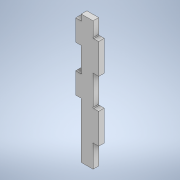
# Autodesk Inventor part: cover
Saved by Autodesk Inventor 2020 (Build 240168000, 168)
## iProperties
Created: 2019-12-19
Part Number: cover
Material: Générique
Document SubType Name: Modeling
Designer: damien
Density: 1 g/cm^3
Appearance: Par défaut
Author: damien
Autodesk Inventor part; units mm, degrees
ref_plane "YZ Plane" through (0, 0, 0) normal (1, 0, 0) x (0, 1, 0)
ref_plane "XZ Plane" through (0, 0, 0) normal (0, 1, 0) x (-1, 0, 0)
ref_plane "XY Plane" through (0, 0, 0) normal (0, 0, 1) x (1, 0, 0)
sketch "Esquisse3" plane through (0, 0, 0) normal (0, 0, 1) x (1, 0, 0)
  line L0 (38, -212.5) -> (-38, -212.5)
  line L1 (-38, -212.5) -> (-38, 212.5)
  line L2 (-38, 212.5) -> (38, 212.5)
  line L3 (38, 212.5) -> (38, -212.5)
  line L4 (38, -212.5) -> (-38, 212.5) construction
  line L5 (-38, -212.5) -> (38, 212.5) construction
  point P0 (0, 0)
  dimension "d20" = 76
  dimension "d21" = 425
  constraints: 12 end point, 2 midpoint, 2 parallel, 1 horizontal, 1 perpendicular
  measures "d20" distance of L0.start L0.end
  measures "d21" distance of L2.end L0.start
extrude "Extrusion3" add sketch "Esquisse3" along normal blind 18.55
sketch "Esquisse4" plane through (0, 0, 18.55) normal (0, 0, 1) x (1, 0, 0)
  line L0 (38, 212.5) -> (19.4, 212.5)
  line L1 (19.4, 212.5) -> (19.4, 162.4)
  line L2 (19.4, 162.4) -> (38, 162.4)
  line L3 (38, 162.4) -> (38, 212.5)
  line L4 (-38, -212.5) -> (38, -212.5) projected
  line L5 (38, -212.5) -> (19.4, -212.5)
  line L6 (19.4, -212.5) -> (19.4, -137.4)
  line L7 (19.4, -137.4) -> (38, -137.4)
  line L8 (38, -137.4) -> (38, -212.5)
  line L9 (38, -37.6) -> (19.4, -37.6)
  line L10 (19.4, -37.6) -> (19.4, 62.6)
  line L11 (19.4, 62.6) -> (38, 62.6)
  line L12 (38, 62.6) -> (38, -37.6)
  point P0 (0, 0)
  dimension "d24" = 75.1
  dimension "d25" = 50.1
  dimension "d27" = 100.2
  dimension "d29" = 99.8
  dimension "d30" = 99.8
  dimension "d31" = 18.6
  constraints: 24 end point, 6 parallel, 3 horizontal, 3 perpendicular, 2 collinear, 1 point on line
  measures "d24" distance of L5.end L6.end
  measures "d25" distance of L0.end L1.end
  measures "d27" distance of L9.end L10.end
  measures "d29" distance between parallel lines of L7 L9
  measures "d30" distance between parallel lines of L2 L11
  measures "d31" distance between parallel lines of L12 L10
extrude "Extrusion4" cut sketch "Esquisse4" against normal blind 18.55
sketch "Esquisse5" plane through (0, 0, 18.55) normal (0, 0, 1) x (1, 0, 0)
  line L0 (19.4, 212.5) -> (-38, 212.5) projected
  line L1 (-38, 212.5) -> (-19.45, 212.5)
  line L2 (-19.45, 212.5) -> (-19.45, 192.4)
  line L3 (-19.45, 192.4) -> (-38, 192.4)
  line L4 (-38, 192.4) -> (-38, 212.5)
  line L5 (-38, 212.5) -> (-38, -212.5) projected
  line L6 (-38, 122.5) -> (-19.45, 122.5)
  line L7 (-19.45, 122.5) -> (-19.45, 41)
  line L8 (-19.45, 41) -> (-38, 41)
  line L9 (-38, 41) -> (-38, 122.5)
  line L10 (-38, -28.9) -> (-19.45, -28.9)
  line L11 (-19.45, -28.9) -> (-19.45, -212.5)
  line L12 (-19.45, -212.5) -> (-38, -212.5)
  line L13 (-38, -212.5) -> (-38, -28.9)
  line L14 (-38, -212.5) -> (19.4, -212.5) projected
  point P0 (0, 0)
  point P1 (-38, 41)
  dimension "d34" = 20.1
  dimension "d35" = 18.55
  dimension "d37" = 69.9
  dimension "d38" = 81.5
  dimension "d39" = 69.9
  constraints: 24 end point, 6 parallel, 3 collinear, 3 horizontal, 3 perpendicular, 2 point on line
  measures "d34" distance of L3.end L0.end
  measures "d35" distance from line of L2 L3.end
  measures "d37" distance between parallel lines of L6 L3
  measures "d38" distance of L6.end L7.end
  measures "d39" distance between parallel lines of L10 L8
extrude "Extrusion5" cut sketch "Esquisse5" against normal blind 18.55
sketch "Esquisse6" plane through (0, 0, 18.55) normal (0, 0, 1) x (1, 0, 0)
  circle A0 centre (-20.5708, 193.5208) radius 1.585
  circle A1 centre (20.5208, 163.5208) radius 1.585
  circle A2 centre (-20.5708, 121.3792) radius 1.585
  circle A3 centre (20.5208, 61.4792) radius 1.585
  circle A4 centre (-20.5708, 42.1208) radius 1.585
  circle A5 centre (20.5208, -36.4792) radius 1.585
  circle A6 centre (-20.5708, -30.0208) radius 1.585
  circle A7 centre (20.5208, -138.5208) radius 1.585
  line L0 (-38, 192.4) -> (-19.45, 192.4) projected
  line L1 (-20.5708, 193.5208) -> (-19.45, 192.4) construction
  line L2 (38, 162.4) -> (19.4, 162.4) projected
  line L3 (19.4, 162.4) -> (20.5208, 163.5208) construction
  line L4 (-19.45, 122.5) -> (-38, 122.5) projected
  line L5 (-19.45, 122.5) -> (-20.5708, 121.3792) construction
  line L6 (-20.5708, 42.1208) -> (-19.45, 41) construction
  line L7 (-38, 41) -> (-19.45, 41) projected
  line L8 (19.4, 62.6) -> (20.5208, 61.4792) construction
  line L9 (-19.45, -28.9) -> (-38, -28.9) projected
  line L10 (-19.45, -28.9) -> (-20.5708, -30.0208) construction
  line L11 (-19.45, -28.9) -> (-19.45, -212.5) projected
  line L12 (38, -37.6) -> (19.4, -37.6) projected
  line L13 (19.4, -37.6) -> (20.5208, -36.4792) construction
  line L14 (19.4, -37.6) -> (19.4, 62.6) projected
  line L15 (19.4, -137.4) -> (38, -137.4) projected
  line L16 (19.4, -137.4) -> (20.5208, -138.5208) construction
  point P0 (0, 0)
  dimension "d43" = 3.17
  dimension "d46" = 45
  dimension "d47" = 45
  dimension "d49" = 45
  dimension "d51" = 45
  dimension "d52" = 45
  dimension "d53" = 45
  dimension "d54" = 45
  constraints: 16 end point, 2 point on circle, 1 centre point, 1 point on line, 1 vertical alignment, 22 other
  measures "d46" angle of L0 L1
  measures "d47" angle of L2 L3
  measures "d49" angle of L7 L6
  measures "d51" angle of L11 L10
  measures "d52" angle of L12 L13
  measures "d53" angle of L14 L8
  measures "d54" angle of L15 L16
extrude "Extrusion6" cut sketch "Esquisse6" against normal blind 18.55
